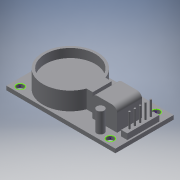
# Autodesk Inventor part: DS1302
Saved by Autodesk Inventor 2016 (Build 200138000, 138)
## iProperties
Created: 2015-11-16
Part Number: DS1302
Material: Generic
Document SubType Name: Modeling
Designer: Jufo
Density: 1 g/cm^3
Appearance: Default
Author: Jufo
Autodesk Inventor part; units mm, degrees
ref_plane "YZ Plane" through (0, 0, 0) normal (1, 0, 0) x (0, 1, 0)
ref_plane "XZ Plane" through (0, 0, 0) normal (0, 1, 0) x (-1, 0, 0)
ref_plane "XY Plane" through (0, 0, 0) normal (0, 0, 1) x (1, 0, 0)
sketch "Sketch1" plane through (0, 0, 0) normal (0, 1, 0) x (-1, 0, 0)
  line L0 (25.7234, 17.199) -> (-18.0766, 17.199)
  line L1 (-18.0766, 17.199) -> (-18.0766, -6.201)
  line L2 (-18.0766, -6.201) -> (25.7234, -6.201)
  line L3 (25.7234, -6.201) -> (25.7234, 17.199)
  point P0 (0, 0)
  dimension "d0" = 43.8
  dimension "d1" = 23.4
  constraints: 8 end point, 2 parallel, 1 horizontal, 1 perpendicular
  measures "d0" distance of L2.end L1.end
  measures "d1" distance of L1.end L0.end
extrude "Extrusion1" add sketch "Sketch1" along normal blind 1.6
sketch "Sketch2" plane through (0, 1.6, 0) normal (0, 1, 0) x (1, 0, 0)
  line L0 (18.0766, -17.199) -> (18.0766, 6.201) projected
  line L1 (14.9766, -11.799) -> (14.9766, 1.001)
  line L2 (-25.7234, -17.199) -> (18.0766, -17.199) projected
  line L3 (14.9766, -11.799) -> (17.4766, -11.799)
  line L4 (17.4766, -11.799) -> (17.4766, 1.001)
  line L5 (17.4766, 1.001) -> (14.9766, 1.001)
  point P0 (0, 0)
  dimension "d6" = 12.8
  dimension "d7" = 0.6
  dimension "d8" = 2.5
  dimension "d9" = 5.4
  constraints: 8 end point, 2 horizontal
  measures "d6" distance of L1.start L1.end
  measures "d7" distance between parallel lines of L0 L4
  measures "d8" distance of L1.start L3.end
  measures "d9" distance between parallel lines of L2 L3
extrude "Extrusion2" add sketch "Sketch2" along normal blind 2.3
sketch "Sketch3" plane through (0, 3.9, 0) normal (0, 1, 0) x (1, 0, 0)
  line L0 (14.9766, -11.799) -> (17.4766, -11.799) projected
  line L1 (16.2266, -11.799) -> (16.2266, -9.669)
  circle A0 centre (16.2266, -9.669) radius 0.35
  circle A1 centre (16.2266, -7.539) radius 0.35
  circle A2 centre (16.2266, -5.409) radius 0.35
  circle A3 centre (16.2266, -3.279) radius 0.35
  circle A4 centre (16.2266, -1.149) radius 0.35
  point P0 (0, 0)
  dimension "d12" = 2.13
  dimension "d13" = 0.7
  dimension "d14" = 0.7
  dimension "d15" = 0.7
  dimension "d16" = 0.7
  dimension "d17" = 0.7
  dimension "d19" = 2.13
  dimension "d20" = 2.13
  dimension "d21" = 2.13
  dimension "d22" = 2.13
  constraints: 5 centre point, 2 end point, 1 coincident, 1 midpoint, 1 vertical
  measures "d12" distance of L1.start L1.end
  measures "d13" diameter of A0
  measures "d14" diameter of A1
  measures "d15" diameter of A2
  measures "d16" diameter of A3
  measures "d17" diameter of A4
  measures "d19" distance of A1.centre L1.end
  measures "d20" distance of A2.centre A1.centre
  measures "d21" distance of A2.centre A3.centre
  measures "d22" distance of A3.centre A4.centre
extrude "Extrusion3" add sketch "Sketch3" along normal blind 6
sketch "Sketch4" plane through (0, 1.6, 0) normal (0, 1, 0) x (1, 0, 0)
  circle A0 centre (-11.7234, -5.499) radius 11
  line L0 (-25.7234, -17.199) -> (18.0766, -17.199) projected
  line L1 (18.0766, 6.201) -> (-25.7234, 6.201) projected
  line L2 (-25.7234, 6.201) -> (-25.7234, -17.199) projected
  point P0 (0, 0)
  dimension "d25" = 22
  dimension "d44" = 14
  dimension "d45" = 11.7
  constraints: 1 centre point
  measures "d25" diameter of A0
  measures "d44" distance from line of A0.centre L2
  measures "d45" distance from line of L1 A0.centre
extrude "Extrusion4" add sketch "Sketch4" along normal blind 7.2
sketch "Sketch5" plane through (0, 1.6, 0) normal (0, 1, 0) x (1, 0, 0)
  circle A0 centre (-11.7234, -5.499) radius 11 projected
  line L0 (-1.4006, -1.699) -> (1.0994, -1.699)
  line L1 (1.0994, -1.699) -> (1.0994, -9.299)
  line L2 (1.0994, -9.299) -> (-1.4006, -9.299)
  point P0 (0, 0)
  dimension "d30" = 7.6
  dimension "d31" = 2.5
  dimension "d32" = 2.5
  constraints: 6 end point, 2 perpendicular, 2 point on circle, 1 horizontal
  measures "d30" distance of L0.end L1.end
  measures "d31" distance of L0.start L0.end
  measures "d32" distance of L1.end L2.end
extrude "Extrusion5" add sketch "Sketch5" along normal blind 7.2 contours A0 L0 L1 L2
sketch "Sketch6" plane through (0, 8.8, 0) normal (0, 1, 0) x (1, 0, 0)
  arc A0 (-1.4006, -1.699) -> (-1.4006, -9.299) centre (-11.7234, -5.499) ccw projected
  circle A1 centre (-11.7234, -5.499) radius 10
  point P0 (0, 0)
  dimension "d35" = 20
  constraints: 1 centre point, 1 coincident
  measures "d35" diameter of A1
extrude "Extrusion6" cut sketch "Sketch6" against normal blind 3.5
sketch "Sketch7" plane through (0, 1.6, 0) normal (0, 1, 0) x (1, 0, 0)
  point P0 (0, 0)
sketch "Sketch8" plane through (0, 1.6, 0) normal (0, 1, 0) x (1, 0, 0)
  line L0 (12.8766, -11.299) -> (12.8766, -1.299)
  line L1 (12.8766, -1.299) -> (2.8766, -1.299)
  line L2 (2.8766, -1.299) -> (2.8766, -11.299)
  line L3 (2.8766, -11.299) -> (12.8766, -11.299)
  line L4 (14.9766, 1.001) -> (14.9766, -11.799) projected
  line L5 (18.0766, 6.201) -> (-25.7234, 6.201) projected
  point P0 (0, 0)
  dimension "d38" = 2.1
  dimension "d39" = 10
  dimension "d40" = 10
  dimension "d41" = 7.5
  constraints: 8 end point, 3 perpendicular, 1 vertical
  measures "d38" distance between parallel lines of L4 L0
  measures "d39" distance of L1.end L2.end
  measures "d40" distance of L0.end L1.end
  measures "d41" distance between parallel lines of L5 L1
extrude "Extrusion7" add sketch "Sketch8" along normal blind 8.8
sketch "Sketch10" plane through (0, 1.6, 0) normal (0, 1, 0) x (1, 0, 0)
  circle A0 centre (9.0766, -14.199) radius 1.5
  line L0 (18.0766, -17.199) -> (18.0766, 6.201) projected
  line L1 (-25.7234, -17.199) -> (18.0766, -17.199) projected
  point P0 (0, 0)
  dimension "d46" = 3
  dimension "d47" = 9
  dimension "d48" = 3
  constraints: 1 centre point
  measures "d46" diameter of A0
  measures "d47" distance from line of L0 A0.centre
  measures "d48" distance from line of L1 A0.centre
extrude "Extrusion8" add sketch "Sketch10" along normal blind 8
fillet "Fillet1" radius 2 2 edges at (12.8766, 10.4, 6.299) (2.8766, 10.4, 6.299)
sketch "Sketch11" plane through (0, 1.6, 0) normal (0, 1, 0) x (1, 0, 0)
  circle A0 centre (13.4766, -14.699) radius 1.5
  circle A1 centre (13.4766, 3.701) radius 1.5
  circle A2 centre (-22.7234, 3.701) radius 1.5
  circle A3 centre (-22.7234, -14.699) radius 1.5
  line L0 (-25.7234, 6.201) -> (-25.7234, -17.199) projected
  line L1 (-25.7234, -17.199) -> (18.0766, -17.199) projected
  point P0 (0, 0)
  dimension "d52" = 3
  dimension "d53" = 3
  dimension "d54" = 21.4
  dimension "d55" = 3
  dimension "d56" = 36.2
  dimension "d57" = 3
  dimension "d58" = 3
  dimension "d59" = 3
  dimension "d60" = 18.4
  dimension "d61" = 2.5
  dimension "d62" = 2.5
  dimension "d64" = 36.2
  constraints: 4 centre point
  measures "d52" diameter of A0
  measures "d53" diameter of A1
  measures "d55" diameter of A2
  measures "d56" distance of A1.centre A2.centre
  measures "d57" diameter of A3
  measures "d58" distance from line of L0 A3.centre
  measures "d59" distance from line of L0 A2.centre
  measures "d60" distance of A2.centre A3.centre
  measures "d61" distance from line of L1 A3.centre
  measures "d62" distance from line of L1 A0.centre
  measures "d64" distance of A0.centre A3.centre
extrude "Extrusion9" cut sketch "Sketch11" against normal blind 8
sketch "Sketch12" plane through (0, 1.6, 0) normal (0, 1, 0) x (1, 0, 0)
  circle A0 centre (-22.7234, -14.699) radius 1.5 projected
  circle A1 centre (-22.7234, -14.699) radius 1.5
  circle A2 centre (-22.7234, 3.701) radius 1.5 projected
  circle A3 centre (-22.7234, 3.701) radius 1.5
  circle A4 centre (13.4766, 3.701) radius 1.5 projected
  circle A5 centre (13.4766, 3.701) radius 1.5
  circle A6 centre (13.4766, -14.699) radius 1.5 projected
  circle A7 centre (13.4766, -14.699) radius 1.5
  point P0 (0, 0)
  constraints: 4 centre point, 4 coincident
body "Solid1"
